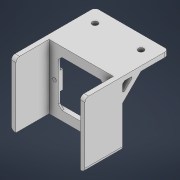
# Autodesk Inventor part: PIR mount
Saved by Autodesk Inventor 2021 (Build 250183000, 183)
## iProperties
Created: 2021-04-15
Part Number: PIR mount
Material: Generic
Document SubType Name: Modeling
Designer: allen
Density: 1 g/cm^3
Appearance: Default
Author: allen
Autodesk Inventor part; units mm, degrees
ref_plane "YZ Plane" through (0, 0, 0) normal (1, 0, 0) x (0, 1, 0)
ref_plane "XZ Plane" through (0, 0, 0) normal (0, 1, 0) x (-1, 0, 0)
sketch "Sketch1" plane through (0, 0, 0) normal (0, 0, 1) x (1, 0, 0)
  line L0 (0, 0) -> (40, 0)
  line L1 (40, 0) -> (40, 35)
  line L2 (40, 35) -> (0, 35)
  line L3 (0, 35) -> (0, 0)
  dimension "d0" = 35
  dimension "d1" = 40
  constraints: 8 end point, 2 parallel, 1 horizontal, 1 perpendicular
  measures "d0" distance of L2.end L0.start
  measures "d1" distance of L0.start L0.end
extrude "Extrusion1" add sketch "Sketch1" along normal blind 2.5
sketch "Sketch2" plane through (0, 0, 2.5) normal (0, 0, 1) x (1, 0, 0)
  line L0 (7.5, 30) -> (32.5, 30)
  line L1 (32.5, 30) -> (32.5, 5)
  line L2 (32.5, 5) -> (7.5, 5)
  line L3 (7.5, 5) -> (7.5, 30)
  line L4 (0, 0) -> (40, 0) projected
  line L5 (0, 35) -> (0, 0) projected
  point P0 (20, 30)
  point P1 (20, 0)
  point P2 (7.5, 17.5)
  point P3 (0, 17.5)
  dimension "d4" = 25
  constraints: 8 end point, 4 midpoint, 2 parallel, 2 perpendicular, 1 horizontal, 1 horizontal alignment, 1 vertical alignment
  measures "d4" distance of L0.end L1.end
extrude "Extrusion2" cut sketch "Sketch2" against normal through all
sketch "Sketch3" plane through (0, 0, 0) normal (0, 0, -1) x (-1, 0, 0)
  line L0 (-5.5, 17.5) -> (-34.5, 17.5)
  line L1 (0, 0) -> (-40, 0) projected
  line L2 (0, 35) -> (0, 0) projected
  point P0 (-20, 17.5)
  point P1 (-20, 0)
  point P2 (0, 17.5)
  dimension "d7" = 29
  constraints: 3 midpoint, 2 end point, 1 horizontal, 1 horizontal alignment, 1 vertical alignment
  measures "d7" distance of L0.start L0.end
hole "Hole1" at (5.5, 17.5, 0) at (34.5, 17.5, 0) direction (0, 0, 1) diameter 2 end through all
sketch "Sketch4" plane through (0, 0, 0) normal (0, 0, -1) x (-1, 0, 0)
  line L0 (-40, 0) -> (-40, 35) projected
  line L1 (0, 35) -> (0, 0) projected
  line L2 (-40, 35) -> (0, 35)
  line L3 (0, 35) -> (0, 32.5)
  line L4 (0, 32.5) -> (-40, 32.5)
  line L5 (-40, 32.5) -> (-40, 35)
  dimension "d15" = 2.5
  constraints: 8 end point, 2 parallel, 1 horizontal, 1 perpendicular, 1 point on line
  measures "d15" distance between parallel lines of L2 L4
extrude "Extrusion3" add sketch "Sketch4" along normal blind 25
fillet "Fillet1" radius 2 4 edges at (40, 0, 1.25) (0, 0, 1.25) (0, 33.75, -25) (40, 33.75, -25)
chamfer "Chamfer1" distance 2 angle 45 4 edges at (7.5, 30, 1.25) (32.5, 30, 1.25) (32.5, 5, 1.25) (7.5, 5, 1.25)
sketch "Sketch5" plane through (40, 2, 0) normal (1, 0, 0) x (0, 0, -1)
  line L0 (0, 30.5) -> (23, 30.5) projected
  line L1 (10, 30.5) -> (0, 20.5)
  line L2 (0, 0) -> (0, 30.5) projected
  line L3 (7.8787, 32.6213) -> (-2.1213, 22.6213)
  point P0 (0, -2)
  point P1 (5.7574, 30.5)
  point P2 (0, 24.7426)
  dimension "d22" = 10
  dimension "d23" = 10
  dimension "d24" = 3
  constraints: 4 end point, 2 point on line, 1 parallel
  measures "d22" distance from line of L2 L1.start
  measures "d23" distance of L1.end L0.start
  measures "d24" distance between parallel lines of L1 L3
extrude "Extrusion4" add sketch "Sketch5" against normal blind 3 contours L0 L1 L2 L3
ref_plane "Work Plane1" through (20, 2, 2.5) normal (1, 0, 0) x (0, 0, -1)
mirror "Mirror1" about plane through (20, 2, 2.5) normal (1, 0, 0) of "Extrusion4"
sketch "Sketch6" plane through (0, 32.5, 0) normal (0, -1, 0) x (1, 0, 0)
  line L0 (7.5, -17.5) -> (32.5, -17.5)
  line L1 (38, -25) -> (2, -25) projected
  point P0 (0, 0)
  point P1 (20, -17.5)
  point P2 (20, -25)
  dimension "d27" = 25
  dimension "d28" = 7.5
  constraints: 2 end point, 2 midpoint, 1 horizontal, 1 vertical alignment
  measures "d27" distance of L0.start L0.end
  measures "d28" distance between parallel lines of L1 L0
hole "Hole2" at (7.5, 32.5, -17.5) at (32.5, 32.5, -17.5) direction (0, 1, 0) diameter 3 end through all
chamfer "Chamfer2" distance 1 angle 45 5 edges at (20, 32.5, 0) (1.5, 32.5, -5.7574) (1.5, 26.7426, 0) (38.5, 32.5, -5.7574) (38.5, 26.7426, 0)
sketch "Sketch7" plane through (0, 0, 0) normal (0, 0, -1) x (-1, 0, 0)
  line L0 (-30.5, 30) -> (-9.5, 30) projected
  line L1 (-30.5, 30) -> (-36.5, 30)
  line L2 (-36.5, 30) -> (-36.5, 5)
  line L3 (-36.5, 5) -> (-30.5, 5)
  line L4 (-32.5, 7) -> (-30.5, 5) projected
  line L5 (-32.5, 7) -> (-32.5, 28) projected
  line L6 (-30.5, 30) -> (-32.5, 28) projected
  line L7 (-32.5, 22.5) -> (-36.5, 22.5)
  line L8 (-32.5, 12.5) -> (-36.5, 12.5)
  line L9 (-34.5, 22.5) -> (-34.5, 12.5) construction
  point P0 (0, 0)
  point P1 (-34.5, 17.5)
  point P2 (-32.5, 17.5)
  dimension "d39" = 6
  dimension "d40" = 10
  constraints: 12 end point, 4 midpoint, 4 perpendicular, 4 point on line, 1 horizontal, 1 horizontal alignment
  measures "d39" distance of L0.start L1.end
  measures "d40" distance of L9.start L9.end
extrude "Extrusion5" cut sketch "Sketch7" against normal blind 1.5 contours L6 L5 L7 L2 L1 | L8 L5 L4 L3 L2
mirror "Mirror2" about plane through (20, 2, 2.5) normal (1, 0, 0) of "Extrusion5"
sketch "Sketch8" plane through (0, 0, 2.5) normal (0, 0, 1) x (1, 0, 0)
  line L0 (0, 35) -> (0, 2) projected
  arc A0 (0, 2) -> (2, 0) centre (2, 2) ccw projected
  line L1 (2, 0) -> (2.5, 0)
  line L2 (2, 0) -> (38, 0) projected
  line L3 (2.5, 0) -> (2.5, 35)
  line L4 (0, 32.5) -> (0, 35) projected
  line L5 (2.5, 35) -> (0, 35)
  point P0 (0, 0)
  dimension "d43" = 0.5
  constraints: 6 end point, 2 perpendicular, 1 point on line
  measures "d43" distance of L1.start L1.end
extrude "Extrusion6" add sketch "Sketch8" along normal blind 18
fillet "Fillet2" radius 2 1 edges at (1.25, 35, 20.5)
mirror "Mirror3" about plane through (20, 2, 2.5) normal (1, 0, 0) of "Extrusion6", "Fillet2"
body "Solid1"
